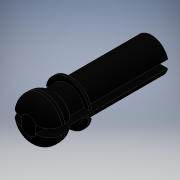
# Autodesk Inventor part: Toggle_Level
Saved by Autodesk Inventor 2016 (Build 200138000, 138)
## iProperties
Created: 2016-04-13
Part Number: Toggle_Level
Material: PC/ABS Plastic
Document SubType Name: Modeling
Designer: agmle
Density: 0.357273 g/cm^3
Appearance: Smooth - Black
Author: agmle
Autodesk Inventor part; units mm, degrees
ref_plane "YZ Plane" through (0, 0, 0) normal (1, 0, 0) x (0, 1, 0)
ref_plane "XZ Plane" through (0, 0, 0) normal (0, 1, 0) x (-1, 0, 0)
ref_plane "XY Plane" through (0, 0, 0) normal (0, 0, 1) x (1, 0, 0)
sketch "Sketch1" plane through (0, 0, 0) normal (0, 1, 0) x (-1, 0, 0)
  line L0 (2.6164, 0.625) -> (1.1164, 0.625)
  line L1 (1.1164, 0.625) -> (1.1164, -0.625)
  line L2 (1.1164, -0.625) -> (2.6164, -0.625)
  line L3 (-2.6164, 0.625) -> (-1.1164, 0.625)
  line L4 (-1.1164, 0.625) -> (-1.1164, -0.625)
  line L5 (-1.1164, -0.625) -> (-2.6164, -0.625)
  line L6 (1.1164, 0) -> (-1.1164, 0) construction
  arc A0 (2.6164, 0.625) -> (-2.6164, 0.625) centre (0, 0) ccw
  arc A1 (-2.6164, -0.625) -> (2.6164, -0.625) centre (0, 0) ccw
  dimension "d1" = 2.69
  dimension "d2" = 2.69
  dimension "d3" = 1.5
  dimension "d4" = 1.25
  constraints: 14 end point, 4 point on circle, 3 midpoint, 2 centre point, 2 coincident, 2 horizontal, 2 parallel, 2 perpendicular, 1 collinear, 1 point on line
  measures "d1" radius of A0
  measures "d2" radius of A1
  measures "d3" distance of L0.start L0.end
  measures "d4" distance of L0.end L1.end
extrude "Extrusion1" add sketch "Sketch1" along normal blind 2.25
sketch "Sketch2" plane through (0, 2.25, 0) normal (0, 1, 0) x (1, 0, 0)
  line L0 (-1.1164, 0.625) -> (-1.1164, -0.625) projected
  line L1 (-1.1164, -0.625) -> (-2.6164, -0.625) projected
  arc A0 (-2.6164, -0.625) -> (2.6164, -0.625) centre (0, 0) ccw construction
  line L2 (2.6164, -0.625) -> (1.1164, -0.625) projected
  line L3 (1.1164, -0.625) -> (1.1164, 0.625) projected
  line L4 (1.1164, 0.625) -> (2.6164, 0.625) projected
  arc A1 (2.6164, 0.625) -> (-2.6164, 0.625) centre (0, 0) ccw construction
  line L5 (-2.6164, 0.625) -> (-1.1164, 0.625) projected
  arc A2 (-3.4437, -0.625) -> (3.4437, -0.625) centre (0, 0) ccw
  arc A3 (3.4437, 0.625) -> (-3.4437, 0.625) centre (0, 0) ccw
  line L6 (-2.6164, -0.625) -> (-3.4437, -0.625)
  arc A4 (2.6164, 0.625) -> (-2.6164, 0.625) centre (0, 0) ccw construction
  line L7 (-2.6164, 0.625) -> (-3.4437, 0.625)
  line L8 (2.6164, 0.625) -> (3.4437, 0.625)
  line L9 (2.6164, -0.625) -> (3.4437, -0.625)
  dimension "d7" = 3.5
  dimension "d8" = 3.5
  constraints: 8 end point, 4 point on circle, 2 centre point, 2 point on line, 1 horizontal, 1 parallel
  measures "d7" radius of A3
  measures "d8" radius of A2
extrude "Extrusion2" add sketch "Sketch2" along normal blind 0.4
sketch "Sketch3" plane through (0, 2.65, 0) normal (0, 1, 0) x (1, 0, 0)
  arc A0 (-2.6164, -0.625) -> (2.6164, -0.625) centre (0, 0) ccw projected
  arc A1 (2.6164, 0.625) -> (-2.6164, 0.625) centre (0, 0) ccw projected
  line L0 (-3.4437, 0.625) -> (-1.1164, 0.625) projected
  line L1 (-1.1164, 0.625) -> (-1.1164, -0.625) projected
  line L2 (-1.1164, -0.625) -> (-3.4437, -0.625) projected
  line L3 (3.4437, -0.625) -> (1.1164, -0.625) projected
  line L4 (1.1164, -0.625) -> (1.1164, 0.625) projected
  line L5 (1.1164, 0.625) -> (3.4437, 0.625) projected
extrude "Extrusion3" add sketch "Sketch3" along normal blind 13
sketch "Sketch4" plane through (0, 0, 0) normal (0, -1, 0) x (1, 0, 0)
  line L0 (-1.1164, -0.625) -> (-1.1164, 0.625) projected
  line L1 (-2.6164, -0.625) -> (-1.1164, -0.625) projected
  arc A0 (-2.6164, -0.625) -> (2.6164, -0.625) centre (0, 0) ccw construction
  line L2 (1.1164, -0.625) -> (2.6164, -0.625) projected
  line L3 (1.1164, 0.625) -> (1.1164, -0.625) projected
  line L4 (2.6164, 0.625) -> (1.1164, 0.625) projected
  arc A1 (2.6164, 0.625) -> (-2.6164, 0.625) centre (0, 0) ccw construction
  line L5 (-1.1164, 0.625) -> (-2.6164, 0.625) projected
  arc A2 (3.3421, 0.625) -> (-3.3421, 0.625) centre (0, 0) ccw
  arc A3 (-3.3421, -0.625) -> (3.3421, -0.625) centre (0, 0) ccw
  line L6 (2.6164, 0.625) -> (3.3421, 0.625)
  line L7 (3.4437, 0.625) -> (2.6164, 0.625) projected
  arc A4 (-2.6164, -0.625) -> (2.6164, -0.625) centre (0, 0) ccw projected
  line L8 (2.6164, -0.625) -> (3.4437, -0.625) projected
  line L9 (-2.6164, -0.625) -> (-3.3421, -0.625)
  line L10 (-3.4437, -0.625) -> (-2.6164, -0.625) projected
  line L11 (-2.6164, 0.625) -> (-3.3421, 0.625)
  line L12 (-2.6164, 0.625) -> (-3.4437, 0.625) projected
  dimension "d13" = 3.4
  dimension "d14" = 3.4
  constraints: 6 end point, 4 point on circle, 4 point on line, 2 centre point
  measures "d13" radius of A2
  measures "d14" radius of A3
extrude "Extrusion4" add sketch "Sketch4" along normal blind 4
fillet "Fillet1" radius 2 2 edges at (0, 0, -3.4) (0, 0, 3.4)
fillet "Fillet2" radius 2 2 edges at (0, -4, -3.4) (0, -4, 3.4)
equation "\"d2\" = d1"
equation "\"d8\" = d7"
equation "\"d14\" = d13"
body "Solid1"
